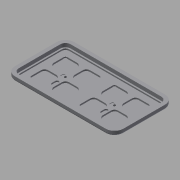
# Autodesk Inventor part: V4 dual
Saved by Autodesk Inventor 2018 (Build 220112000, 112)
## iProperties
Created: 2020-01-08
Part Number: V4 dual
Material: Generic
Document SubType Name: Modeling
Designer: user
Density: 1 g/cm^3
Appearance: Default
Author: user
Autodesk Inventor part; units mm, degrees
ref_plane "YZ Plane" through (0, 0, 0) normal (1, 0, 0) x (0, 1, 0)
ref_plane "XZ Plane" through (0, 0, 0) normal (0, 1, 0) x (-1, 0, 0)
ref_plane "XY Plane" through (0, 0, 0) normal (0, 0, 1) x (1, 0, 0)
sketch "Sketch1" plane through (0, 0, 0) normal (0, 0, 1) x (1, 0, 0)
  line L0 (-62, 40.5) -> (62, 40.5)
  line L1 (74, 28.5) -> (74, -28.5)
  line L2 (62, -40.5) -> (-62, -40.5)
  line L3 (-74, -28.5) -> (-74, 28.5)
  arc A0 (-62, 40.5) -> (-74, 28.5) centre (-62, 28.5) ccw
  arc A1 (74, 28.5) -> (62, 40.5) centre (62, 28.5) ccw
  arc A2 (62, -40.5) -> (74, -28.5) centre (62, -28.5) ccw
  arc A3 (-74, -28.5) -> (-62, -40.5) centre (-62, -28.5) ccw
  line L4 (-62, 28.5) -> (62, -28.5) construction
  point P0 (0, 0)
  point P1 (0, 0)
  dimension "d0" = 12
  dimension "d1" = 81
  dimension "d40" = 148
  constraints: 10 end point, 8 point on circle, 8 tangent, 4 centre point, 3 equal radius, 2 parallel, 1 coincident, 1 horizontal, 1 midpoint, 1 perpendicular
  measures "d0" radius of A0
  measures "d1" distance between parallel lines of L2 L0
  measures "d40" distance between parallel lines of L1 L3
extrude "Extrusion1" add sketch "Sketch1" along normal blind 10.25
sketch "Sketch2" plane through (0, 0, 10.25) normal (0, 0, 1) x (1, 0, 0)
  line L0 (62, 40.5) -> (-62, 40.5) construction
  arc A0 (-62, 40.5) -> (-74, 28.5) centre (-62, 28.5) ccw construction
  line L1 (-74, 28.5) -> (-74, -28.5) construction
  arc A1 (-74, -28.5) -> (-62, -40.5) centre (-62, -28.5) ccw construction
  line L2 (-62, -40.5) -> (62, -40.5) construction
  arc A2 (62, -40.5) -> (74, -28.5) centre (62, -28.5) ccw construction
  line L3 (74, -28.5) -> (74, 28.5) construction
  arc A3 (74, 28.5) -> (62, 40.5) centre (62, 28.5) ccw construction
  line L4 (-62, 35.5) -> (62, 35.5)
  arc A4 (69, 28.5) -> (62, 35.5) centre (62, 28.5) ccw
  line L5 (69, 28.5) -> (69, -28.5)
  arc A5 (62, -35.5) -> (69, -28.5) centre (62, -28.5) ccw
  line L6 (62, -35.5) -> (-62, -35.5)
  arc A6 (-69, -28.5) -> (-62, -35.5) centre (-62, -28.5) ccw
  line L7 (-69, -28.5) -> (-69, 28.5)
  arc A7 (-62, 35.5) -> (-69, 28.5) centre (-62, 28.5) ccw
  point P0 (0, 0)
  dimension "d4" = 5
  constraints: 8 end point, 8 point on circle, 4 centre point, 7 other
  measures "d4" distance between parallel lines of L1 L7
extrude "Extrusion2" cut sketch "Sketch2" against normal blind 5
sketch "Sketch3" plane through (0, 0, 5.25) normal (0, 0, 1) x (1, 0, 0)
  line L0 (-62, 35.5) -> (62, 35.5) construction
  arc A0 (-62, 35.5) -> (-69, 28.5) centre (-62, 28.5) ccw construction
  line L1 (-69, -28.5) -> (-69, 28.5) construction
  arc A1 (-69, -28.5) -> (-62, -35.5) centre (-62, -28.5) ccw construction
  line L2 (62, -35.5) -> (-62, -35.5) construction
  arc A2 (62, -35.5) -> (69, -28.5) centre (62, -28.5) ccw construction
  line L3 (69, 28.5) -> (69, -28.5) construction
  arc A3 (69, 28.5) -> (62, 35.5) centre (62, 28.5) ccw construction
  line L4 (62, 33.5) -> (-62, 33.5)
  arc A4 (-62, 33.5) -> (-67, 28.5) centre (-62, 28.5) ccw
  line L5 (-67, 28.5) -> (-67, -28.5)
  arc A5 (-67, -28.5) -> (-62, -33.5) centre (-62, -28.5) ccw
  line L6 (-62, -33.5) -> (62, -33.5)
  arc A6 (62, -33.5) -> (67, -28.5) centre (62, -28.5) ccw
  line L7 (67, -28.5) -> (67, 28.5)
  arc A7 (67, 28.5) -> (62, 33.5) centre (62, 28.5) ccw
  point P0 (0, 0)
  dimension "d7" = 2
  constraints: 8 end point, 8 point on circle, 4 centre point, 7 other
  measures "d7" distance between parallel lines of L0 L4
extrude "Extrusion3" cut sketch "Sketch3" against normal blind 1.75
chamfer "Chamfer1" distance 9 angle 30 8 edges at (0, 40.5, 0) (70.4853, 36.9853, 0) (74, 0, 0) (70.4853, -36.9853, 0) (0, -40.5, 0) (-70.4853, -36.9853, 0) (-74, 0, 0) (-70.4853, 36.9853, 0) measured on face at (70.1317, 36.6317, 0) measured on face at (0, 40, 0) measured on face at (-70.1317, -36.6317, 0) measured on face at (0, -40, 0) measured on face at (-73.5, 0, 0) measured on face at (70.1317, -36.6317, 0) measured on face at (73.5, 0, 0) measured on face at (-70.1317, 36.6317, 0)
sketch "Sketch5" plane through (0, 0, 0) normal (0, 0, -1) x (-1, 0, 0)
  line L0 (24.75, 3.75) -> (13.75, 3.75)
  line L1 (8.75, 8.75) -> (8.75, 22.0251)
  line L2 (11.4749, 24.75) -> (24.75, 24.75)
  line L3 (29.75, 19.75) -> (29.75, 8.75)
  arc A0 (8.75, 8.75) -> (13.75, 3.75) centre (13.75, 8.75) ccw
  arc A1 (29.75, 19.75) -> (24.75, 24.75) centre (24.75, 19.75) ccw
  arc A2 (24.75, 3.75) -> (29.75, 8.75) centre (24.75, 8.75) ccw
  line L4 (50.752, -17.252) -> (24.75, 8.75) construction
  line L5 (24.75, 24.25) -> (11.4749, 24.25)
  line L6 (9.25, 22.0251) -> (9.25, 8.75)
  arc A3 (9.25, 8.75) -> (13.75, 4.25) centre (13.75, 8.75) ccw
  line L7 (13.75, 4.25) -> (24.75, 4.25)
  arc A4 (24.75, 4.25) -> (29.25, 8.75) centre (24.75, 8.75) ccw
  line L8 (29.25, 8.75) -> (29.25, 19.75)
  arc A5 (29.25, 19.75) -> (24.75, 24.25) centre (24.75, 19.75) ccw
  line L9 (-12.252, 45.752) -> (13.75, 19.75) construction
  line L10 (24.75, 24.25) -> (24.75, 4.25) construction
  line L11 (9.25, 8.75) -> (29.25, 8.75) construction
  line L12 (24.75, 24.25) -> (24.75, 24.75) construction
  line L13 (9.25, 8.75) -> (8.75, 8.75) construction
  line L14 (24.75, 19.75) -> (13.75, 19.75) construction
  line L15 (13.75, 8.75) -> (13.75, 19.75) construction
  arc A6 (11.2249, 24.5) -> (11.4749, 24.25) centre (11.4749, 24.5) ccw
  arc A7 (11.4749, 24.75) -> (11.2249, 24.5) centre (11.4749, 24.5) ccw
  arc A8 (9.25, 22.0251) -> (9, 21.7751) centre (9, 22.0251) ccw construction
  arc A9 (9, 21.7751) -> (8.75, 22.0251) centre (9, 22.0251) ccw construction
  line L16 (10.2374, 23.2626) -> (11.2981, 24.3232) construction
  line L17 (10.2374, 23.2626) -> (9.1768, 22.2019) construction
  arc A10 (-62, 31.5) -> (-65, 28.5) centre (-62, 28.5) ccw construction
  arc A11 (9.25, 22.0251) -> (8.75, 22.0251) centre (9, 22.0251) ccw
  line L18 (29.75, -8.75) -> (29.75, -19.75)
  line L19 (24.75, -4.25) -> (13.75, -4.25)
  line L20 (29.25, -19.75) -> (29.25, -8.75)
  line L21 (9.25, -8.75) -> (29.25, -8.75) construction
  line L22 (24.75, -24.25) -> (24.75, -4.25) construction
  arc A12 (13.75, -4.25) -> (9.25, -8.75) centre (13.75, -8.75) ccw
  line L23 (24.75, -19.75) -> (13.75, -19.75) construction
  line L24 (13.75, -8.75) -> (13.75, -19.75) construction
  line L25 (10.2374, -23.2626) -> (11.2981, -24.3232) construction
  line L26 (9.25, -8.75) -> (9.25, -22.0251)
  line L27 (8.75, -22.0251) -> (8.75, -8.75)
  line L28 (9.25, -8.75) -> (8.75, -8.75) construction
  arc A13 (13.75, -3.75) -> (8.75, -8.75) centre (13.75, -8.75) ccw
  line L29 (13.75, -3.75) -> (24.75, -3.75)
  arc A14 (29.75, -8.75) -> (24.75, -3.75) centre (24.75, -8.75) ccw
  arc A15 (29.25, -8.75) -> (24.75, -4.25) centre (24.75, -8.75) ccw
  line L30 (24.75, -24.75) -> (11.4749, -24.75)
  line L31 (11.4749, -24.25) -> (24.75, -24.25)
  line L32 (24.75, -24.25) -> (24.75, -24.75) construction
  arc A16 (24.75, -24.25) -> (29.25, -19.75) centre (24.75, -19.75) ccw
  arc A17 (24.75, -24.75) -> (29.75, -19.75) centre (24.75, -19.75) ccw
  arc A18 (8.75, -22.0251) -> (9, -22.2751) centre (9, -22.0251) ccw
  arc A19 (9, -22.2751) -> (9.25, -22.0251) centre (9, -22.0251) ccw
  line L33 (10.2374, -23.2626) -> (9.1768, -22.2019) construction
  arc A20 (11.7249, -24.5) -> (11.4749, -24.75) centre (11.4749, -24.5) ccw construction
  arc A21 (11.4749, -24.25) -> (11.7249, -24.5) centre (11.4749, -24.5) ccw construction
  arc A22 (11.4749, -24.25) -> (11.4749, -24.75) centre (11.4749, -24.5) ccw
  line L34 (42.25, -3.75) -> (53.25, -3.75)
  line L35 (37.75, -8.75) -> (37.75, -19.75)
  line L36 (53.25, -4.25) -> (42.25, -4.25)
  line L37 (42.25, -24.25) -> (42.25, -4.25) construction
  line L38 (57.75, -8.75) -> (37.75, -8.75) construction
  arc A23 (37.75, -19.75) -> (42.25, -24.25) centre (42.25, -19.75) ccw
  line L39 (53.25, -8.75) -> (53.25, -19.75) construction
  line L40 (42.25, -19.75) -> (53.25, -19.75) construction
  line L41 (56.7626, -23.2626) -> (57.8232, -22.2019) construction
  line L42 (42.25, -24.25) -> (55.5251, -24.25)
  line L43 (55.5251, -24.75) -> (42.25, -24.75)
  line L44 (42.25, -24.25) -> (42.25, -24.75) construction
  arc A24 (37.25, -19.75) -> (42.25, -24.75) centre (42.25, -19.75) ccw
  line L45 (37.25, -19.75) -> (37.25, -8.75)
  arc A25 (42.25, -3.75) -> (37.25, -8.75) centre (42.25, -8.75) ccw
  arc A26 (42.25, -4.25) -> (37.75, -8.75) centre (42.25, -8.75) ccw
  line L46 (58.25, -8.75) -> (58.25, -22.0251)
  line L47 (57.75, -22.0251) -> (57.75, -8.75)
  line L48 (57.75, -8.75) -> (58.25, -8.75) construction
  arc A27 (57.75, -8.75) -> (53.25, -4.25) centre (53.25, -8.75) ccw
  arc A28 (58.25, -8.75) -> (53.25, -3.75) centre (53.25, -8.75) ccw
  arc A29 (55.5251, -24.75) -> (55.7751, -24.5) centre (55.5251, -24.5) ccw
  arc A30 (55.7751, -24.5) -> (55.5251, -24.25) centre (55.5251, -24.5) ccw
  line L49 (56.7626, -23.2626) -> (55.7019, -24.3232) construction
  arc A31 (58, -21.7751) -> (58.25, -22.0251) centre (58, -22.0251) ccw construction
  arc A32 (57.75, -22.0251) -> (58, -21.7751) centre (58, -22.0251) ccw construction
  arc A33 (57.75, -22.0251) -> (58.25, -22.0251) centre (58, -22.0251) ccw
  line L50 (37.25, 8.75) -> (37.25, 19.75)
  line L51 (42.25, 4.25) -> (53.25, 4.25)
  line L52 (37.75, 19.75) -> (37.75, 8.75)
  line L53 (57.75, 8.75) -> (37.75, 8.75) construction
  line L54 (42.25, 24.25) -> (42.25, 4.25) construction
  arc A34 (53.25, 4.25) -> (57.75, 8.75) centre (53.25, 8.75) ccw
  line L55 (42.25, 19.75) -> (53.25, 19.75) construction
  line L56 (53.25, 8.75) -> (53.25, 19.75) construction
  line L57 (56.7626, 23.2626) -> (55.7019, 24.3232) construction
  line L58 (57.75, 8.75) -> (57.75, 22.0251)
  line L59 (58.25, 22.0251) -> (58.25, 8.75)
  line L60 (57.75, 8.75) -> (58.25, 8.75) construction
  arc A35 (53.25, 3.75) -> (58.25, 8.75) centre (53.25, 8.75) ccw
  line L61 (53.25, 3.75) -> (42.25, 3.75)
  arc A36 (37.25, 8.75) -> (42.25, 3.75) centre (42.25, 8.75) ccw
  arc A37 (37.75, 8.75) -> (42.25, 4.25) centre (42.25, 8.75) ccw
  line L62 (42.25, 24.75) -> (55.5251, 24.75)
  line L63 (55.5251, 24.25) -> (42.25, 24.25)
  line L64 (42.25, 24.25) -> (42.25, 24.75) construction
  arc A38 (42.25, 24.25) -> (37.75, 19.75) centre (42.25, 19.75) ccw
  arc A39 (42.25, 24.75) -> (37.25, 19.75) centre (42.25, 19.75) ccw
  arc A40 (58.25, 22.0251) -> (58, 22.2751) centre (58, 22.0251) ccw
  arc A41 (58, 22.2751) -> (57.75, 22.0251) centre (58, 22.0251) ccw
  line L65 (56.7626, 23.2626) -> (57.8232, 22.2019) construction
  arc A42 (55.2751, 24.5) -> (55.5251, 24.75) centre (55.5251, 24.5) ccw construction
  arc A43 (55.5251, 24.25) -> (55.2751, 24.5) centre (55.5251, 24.5) ccw construction
  arc A44 (55.5251, 24.25) -> (55.5251, 24.75) centre (55.5251, 24.5) ccw
  line L66 (33.5, 0) -> (0, 0)
  line L67 (58.25, -15.3876) -> (65, -15.3876) construction
  line L68 (65, 28.5) -> (65, -28.5) construction
  line L69 (48.8876, -24.75) -> (48.8876, -31.5) construction
  line L70 (62, -31.5) -> (-62, -31.5) construction
  point P0 (11.2249, 24.75)
  point P1 (8.75, 21.7751)
  point P2 (9.25, 21.7751)
  point P3 (11.2249, 24.25)
  point P4 (9.25, -22.2751)
  point P5 (8.75, -22.2751)
  point P6 (11.7249, -24.75)
  point P7 (11.7249, -24.25)
  point P8 (55.7751, -24.25)
  point P9 (55.7751, -24.75)
  point P10 (58.25, -21.7751)
  point P11 (57.75, -21.7751)
  point P12 (57.75, 22.2751)
  point P13 (58.25, 22.2751)
  point P14 (55.2751, 24.75)
  point P15 (55.2751, 24.25)
  dimension "d23" = 0.5
  dimension "d24" = 5
  dimension "d25" = 20
  dimension "d26" = 0.25
  dimension "d27" = 3
  dimension "d32" = 360
  dimension "d41" = 7.5
  constraints: 138 end point, 96 point on circle, 44 centre point, 27 point on line, 11 tangent, 7 perpendicular, 6 equal length, 4 horizontal, 4 parallel, 3 collinear, 3 equal radius, 2 midpoint, 2 vertical, 1 coincident, 315 other
  measures "d23" distance between parallel lines of L0 L7
  measures "d24" radius of A0
  measures "d25" distance between parallel lines of L8 L6
  measures "d26" radius of A6
  measures "d27" distance of L17.end L16.end
  measures "d41" distance between parallel lines of L50 L3
extrude "Extrusion4" cut sketch "Sketch5" against normal through all
fillet "Fillet2" radius 2 16 edges at (70.4853, 36.9853, 5.1962) (74, 0, 5.1962) (70.4853, -36.9853, 5.1962) (0, -40.5, 5.1962) (-70.4853, -36.9853, 5.1962) (-74, 0, 5.1962) (-70.4853, 36.9853, 5.1962) (0, 40.5, 5.1962) (-64.1213, 30.6213, 0) (-65, 0, 0) (-64.1213, -30.6213, 0) (0, -31.5, 0) (64.1213, -30.6213, 0) (65, 0, 0) (64.1213, 30.6213, 0) (0, 31.5, 0)
sketch "Sketch7" plane through (0, 0, 3.5) normal (0, 0, 1) x (1, 0, 0)
  line L0 (-37.25, -8.75) -> (-37.25, -19.75) projected
  arc A0 (-42.25, -24.75) -> (-37.25, -19.75) centre (-42.25, -19.75) ccw projected
  line L1 (-42.25, -24.75) -> (-55.5251, -24.75) projected
  arc A1 (-55.5251, -24.25) -> (-55.5251, -24.75) centre (-55.5251, -24.5) ccw projected
  line L2 (-55.5251, -24.25) -> (-42.25, -24.25) projected
  arc A2 (-42.25, -24.25) -> (-37.75, -19.75) centre (-42.25, -19.75) ccw projected
  line L3 (-37.75, -19.75) -> (-37.75, -8.75) projected
  arc A3 (-37.75, -8.75) -> (-42.25, -4.25) centre (-42.25, -8.75) ccw projected
  line L4 (-42.25, -4.25) -> (-53.25, -4.25) projected
  arc A4 (-53.25, -4.25) -> (-57.75, -8.75) centre (-53.25, -8.75) ccw projected
  line L5 (-57.75, -8.75) -> (-57.75, -22.0251) projected
  arc A5 (-58.25, -22.0251) -> (-57.75, -22.0251) centre (-58, -22.0251) ccw projected
  line L6 (-58.25, -22.0251) -> (-58.25, -8.75) projected
  arc A6 (-53.25, -3.75) -> (-58.25, -8.75) centre (-53.25, -8.75) ccw projected
  line L7 (-53.25, -3.75) -> (-42.25, -3.75) projected
  arc A7 (-37.25, -8.75) -> (-42.25, -3.75) centre (-42.25, -8.75) ccw projected
  line L8 (-11.4749, 24.25) -> (-24.75, 24.25) projected
  arc A8 (-24.75, 24.25) -> (-29.25, 19.75) centre (-24.75, 19.75) ccw projected
  line L9 (-29.25, 19.75) -> (-29.25, 8.75) projected
  arc A9 (-29.25, 8.75) -> (-24.75, 4.25) centre (-24.75, 8.75) ccw projected
  line L10 (-24.75, 4.25) -> (-13.75, 4.25) projected
  arc A10 (-13.75, 4.25) -> (-9.25, 8.75) centre (-13.75, 8.75) ccw projected
  line L11 (-9.25, 8.75) -> (-9.25, 22.0251) projected
  arc A11 (-8.75, 22.0251) -> (-9.25, 22.0251) centre (-9, 22.0251) ccw projected
  line L12 (-8.75, 22.0251) -> (-8.75, 8.75) projected
  arc A12 (-13.75, 3.75) -> (-8.75, 8.75) centre (-13.75, 8.75) ccw projected
  line L13 (-13.75, 3.75) -> (-24.75, 3.75) projected
  arc A13 (-29.75, 8.75) -> (-24.75, 3.75) centre (-24.75, 8.75) ccw projected
  line L14 (-29.75, 8.75) -> (-29.75, 19.75) projected
  arc A14 (-24.75, 24.75) -> (-29.75, 19.75) centre (-24.75, 19.75) ccw projected
  line L15 (-24.75, 24.75) -> (-11.4749, 24.75) projected
  arc A15 (-11.4749, 24.25) -> (-11.4749, 24.75) centre (-11.4749, 24.5) ccw projected
  line L16 (-24.75, -3.75) -> (-13.75, -3.75) projected
  arc A16 (-8.75, -8.75) -> (-13.75, -3.75) centre (-13.75, -8.75) ccw projected
  line L17 (-8.75, -8.75) -> (-8.75, -22.0251) projected
  arc A17 (-9.25, -22.0251) -> (-8.75, -22.0251) centre (-9, -22.0251) ccw projected
  line L18 (-9.25, -22.0251) -> (-9.25, -8.75) projected
  arc A18 (-9.25, -8.75) -> (-13.75, -4.25) centre (-13.75, -8.75) ccw projected
  line L19 (-13.75, -4.25) -> (-24.75, -4.25) projected
  arc A19 (-24.75, -4.25) -> (-29.25, -8.75) centre (-24.75, -8.75) ccw projected
  line L20 (-29.25, -8.75) -> (-29.25, -19.75) projected
  arc A20 (-29.25, -19.75) -> (-24.75, -24.25) centre (-24.75, -19.75) ccw projected
  line L21 (-24.75, -24.25) -> (-11.4749, -24.25) projected
  arc A21 (-11.4749, -24.75) -> (-11.4749, -24.25) centre (-11.4749, -24.5) ccw projected
  line L22 (-11.4749, -24.75) -> (-24.75, -24.75) projected
  arc A22 (-29.75, -19.75) -> (-24.75, -24.75) centre (-24.75, -19.75) ccw projected
  line L23 (-29.75, -19.75) -> (-29.75, -8.75) projected
  arc A23 (-24.75, -3.75) -> (-29.75, -8.75) centre (-24.75, -8.75) ccw projected
  line L24 (-42.25, 3.75) -> (-53.25, 3.75) projected
  arc A24 (-58.25, 8.75) -> (-53.25, 3.75) centre (-53.25, 8.75) ccw projected
  line L25 (-58.25, 8.75) -> (-58.25, 22.0251) projected
  arc A25 (-57.75, 22.0251) -> (-58.25, 22.0251) centre (-58, 22.0251) ccw projected
  line L26 (-57.75, 22.0251) -> (-57.75, 8.75) projected
  arc A26 (-57.75, 8.75) -> (-53.25, 4.25) centre (-53.25, 8.75) ccw projected
  line L27 (-53.25, 4.25) -> (-42.25, 4.25) projected
  arc A27 (-42.25, 4.25) -> (-37.75, 8.75) centre (-42.25, 8.75) ccw projected
  line L28 (-37.75, 8.75) -> (-37.75, 19.75) projected
  arc A28 (-37.75, 19.75) -> (-42.25, 24.25) centre (-42.25, 19.75) ccw projected
  line L29 (-42.25, 24.25) -> (-55.5251, 24.25) projected
  arc A29 (-55.5251, 24.75) -> (-55.5251, 24.25) centre (-55.5251, 24.5) ccw projected
  line L30 (-55.5251, 24.75) -> (-42.25, 24.75) projected
  arc A30 (-37.25, 19.75) -> (-42.25, 24.75) centre (-42.25, 19.75) ccw projected
  line L31 (-37.25, 19.75) -> (-37.25, 8.75) projected
  arc A31 (-42.25, 3.75) -> (-37.25, 8.75) centre (-42.25, 8.75) ccw projected
  line L32 (-62, 33.5) -> (62, 33.5) projected
  arc A32 (-62, 33.5) -> (-67, 28.5) centre (-62, 28.5) ccw projected
  line L33 (-67, -28.5) -> (-67, 28.5) projected
  arc A33 (-67, -28.5) -> (-62, -33.5) centre (-62, -28.5) ccw projected
  line L34 (62, -33.5) -> (-62, -33.5) projected
  arc A34 (62, -33.5) -> (67, -28.5) centre (62, -28.5) ccw projected
  line L35 (67, 28.5) -> (67, -28.5) projected
  arc A35 (67, 28.5) -> (62, 33.5) centre (62, 28.5) ccw projected
  arc A36 (-58.25, -22.0251) -> (-55.5251, -24.75) centre (-55.5251, -22.0251) ccw
  arc A37 (-55.5251, 24.75) -> (-58.25, 22.0251) centre (-55.5251, 22.0251) ccw
  arc A38 (-11.4749, 24.25) -> (-11.4749, 24.75) centre (-11.4749, 24.5) ccw projected
  arc A39 (-8.75, 22.0251) -> (-11.4749, 24.75) centre (-11.4749, 22.0251) ccw
  line L36 (-11.4749, -24.75) -> (-24.75, -24.75) projected
  arc A40 (-11.4749, -24.75) -> (-8.75, -22.0251) centre (-11.4749, -22.0251) ccw
  point P0 (0, 0)
  constraints: 8 point on circle, 4 centre point, 4 tangent
extrude "Extrusion6" cut sketch "Sketch7" against normal blind 1.5 contours L0 A0 L1 A1 L2 A2 L3 A3 L4 A4 L5 A5 L6 A6 L7 A7 | A36 A5 L5 A4 L4 A3 L3 A2 L2 A1 | A15 A39 A11 L11 A10 L10 A9 L9 A8 L8 | L8 A8 L9 A9 L10 A10 L11 A11 L12 A12 L13 A13 L14 A14 L15 A15 | L16 A16 L17 A17 L18 A18 L19 A19 L20 A20 L21 A21 L22 A22 L23 A23 | A40 A21 L21 A20 L20 A19 L19 A18 L18 A17 | L24 A24 L25 A25 L26 A26 L27 A27 L28 A28 L29 A29 L30 A30 L31 A31 | A37 A29 L29 A28 L28 A27 L27 A26 L26 A25
sketch "Sketch8" plane through (0, 0, 0) normal (0, 0, -1) x (-1, 0, 0)
  arc A0 (42.25, -4.25) -> (37.75, -8.75) centre (42.25, -8.75) ccw construction
  arc A1 (24.75, 4.25) -> (29.25, 8.75) centre (24.75, 8.75) ccw construction
  line L0 (42.25, -8.75) -> (24.75, 8.75) construction
  point P0 (0, 0)
  point P1 (33.5, 0)
  constraints: 2 end point, 1 midpoint
hole "Hole1" at (-33.5, 0, 0) direction (0, 0, 1) diameter 3.2 end through all counterbore diameter 5.7 counterbore depth 2.7
sketch "Sketch10" plane through (0, 0, 3.5) normal (0, 0, 1) x (1, 0, 0)
  line L0 (-37.961, -2.5) -> (-36.461, -2.5)
  line L1 (-35.711, -1.75) -> (-35.711, 1.75)
  line L2 (-36.461, 2.5) -> (-37.961, 2.5)
  line L3 (-38.711, 1.75) -> (-38.711, -1.75)
  line L4 (-33.5, -16.4884) -> (-33.5, -11.4084) construction
  line L5 (-31.25, -16.4884) -> (-31.25, -11.4084)
  line L6 (-35.75, -11.4084) -> (-35.75, -16.4884)
  arc A0 (-35.75, -16.4884) -> (-31.25, -16.4884) centre (-33.5, -16.4884) ccw
  arc A1 (-31.25, -11.4084) -> (-35.75, -11.4084) centre (-33.5, -11.4084) ccw
  circle A2 centre (-33.5, 0) radius 1.6 construction
  line L7 (-35.75, -13.9484) -> (-35.75, -12.4484) construction
  line L8 (-31.25, -13.9484) -> (-31.25, -15.4484) construction
  arc A3 (-37.961, 2.5) -> (-38.711, 1.75) centre (-37.961, 1.75) ccw
  arc A4 (-38.711, -1.75) -> (-37.961, -2.5) centre (-37.961, -1.75) ccw
  arc A5 (-36.461, -2.5) -> (-35.711, -1.75) centre (-36.461, -1.75) ccw
  arc A6 (-35.711, 1.75) -> (-36.461, 2.5) centre (-36.461, 1.75) ccw
  line L9 (-37.961, -1.75) -> (-33.5, 0) construction
  line L10 (-33.5, 0) -> (-37.961, 1.75) construction
  line L11 (-37.25, -8.75) -> (-37.25, -19.75) construction
  point P0 (-38.711, -2.5)
  point P1 (-35.711, 2.5)
  point P2 (-38.711, 2.5)
  point P3 (-33.5, -13.9484)
  dimension "d70" = 5
  dimension "d71" = 3
  dimension "d73" = 5.08
  dimension "d76" = 0.75
  dimension "d84" = 13.9484
  dimension "d85" = 2.211
  dimension "d86" = 4.5
  constraints: 24 end point, 12 point on circle, 12 tangent, 7 point on line, 6 centre point, 5 parallel, 3 equal radius, 3 midpoint, 2 coincident, 2 equal length, 1 perpendicular
  measures "d70" distance of point (-38.711, 2.5) point (-38.711, -2.5)
  measures "d71" distance of point (-35.711, 2.5) point (-38.711, 2.5)
  measures "d73" distance of L5.start L5.end
  measures "d76" radius of A3
  measures "d84" distance of L9.end point (-33.5, -13.948)
  measures "d85" distance from line of L9.end L1
  measures "d86" distance between parallel lines of L5 L6
extrude "Extrusion7" cut sketch "Sketch10" against normal blind 0.64 contours A4 L3 A3 L2 A6 L1 A5 L0
extrude "Extrusion8" cut sketch "Sketch10" against normal blind 1.75 contours A0 L6 A1 L5
sketch "Sketch9" plane through (0, 0, 0) normal (0, 0, -1) x (-1, 0, 0)
  arc A0 (29.25, 19.75) -> (24.75, 24.25) centre (24.75, 19.75) ccw construction
  circle A1 centre (33.5, 0) radius 1.6 construction
  arc A2 (9.25, 8.75) -> (13.75, 4.25) centre (13.75, 8.75) ccw construction
  line L0 (24.75, 19.75) -> (13.75, 8.75) construction
  circle A3 centre (19.25, 14.25) radius 2
  circle A4 centre (16.4216, 11.4216) radius 2
  circle A5 centre (17.25, 10.7859) radius 2
  circle A6 centre (18.2147, 10.3863) radius 2
  circle A7 centre (19.25, 10.25) radius 2
  circle A8 centre (20.2853, 10.3863) radius 2
  circle A9 centre (21.25, 10.7859) radius 2
  circle A10 centre (22.0784, 11.4216) radius 2
  circle A11 centre (22.7141, 12.25) radius 2
  circle A12 centre (23.1137, 13.2147) radius 2
  circle A13 centre (23.25, 14.25) radius 2
  circle A14 centre (23.1137, 15.2853) radius 2
  circle A15 centre (22.7141, 16.25) radius 2
  circle A16 centre (22.0784, 17.0784) radius 2
  circle A17 centre (21.25, 17.7141) radius 2
  circle A18 centre (20.2853, 18.1137) radius 2
  circle A19 centre (19.25, 18.25) radius 2
  circle A20 centre (18.2147, 18.1137) radius 2
  circle A21 centre (17.25, 17.7141) radius 2
  circle A22 centre (16.4216, 17.0784) radius 2
  circle A23 centre (15.7859, 16.25) radius 2
  circle A24 centre (15.3863, 15.2853) radius 2
  circle A25 centre (15.25, 14.25) radius 2
  circle A26 centre (15.3863, 13.2147) radius 2
  circle A27 centre (15.7859, 12.25) radius 2
  circle A28 centre (22.7141, -12.25) radius 2
  circle A29 centre (23.1137, -13.2147) radius 2
  circle A30 centre (23.1137, -15.2853) radius 2
  circle A31 centre (22.7141, -16.25) radius 2
  circle A32 centre (23.25, -14.25) radius 2
  circle A33 centre (15.3863, -13.2147) radius 2
  circle A34 centre (15.25, -14.25) radius 2
  circle A35 centre (15.3863, -15.2853) radius 2
  circle A36 centre (19.25, -18.25) radius 2
  circle A37 centre (18.2147, -18.1137) radius 2
  circle A38 centre (15.7859, -16.25) radius 2
  circle A39 centre (16.4216, -17.0784) radius 2
  circle A40 centre (17.25, -17.7141) radius 2
  circle A41 centre (22.0784, -11.4216) radius 2
  circle A42 centre (21.25, -10.7859) radius 2
  line L1 (13.75, -8.75) -> (24.75, -19.75) construction
  circle A43 centre (19.25, -14.25) radius 2
  circle A44 centre (19.25, -10.25) radius 2
  circle A45 centre (15.7859, -12.25) radius 2
  circle A46 centre (18.2147, -10.3863) radius 2
  circle A47 centre (16.4216, -11.4216) radius 2
  circle A48 centre (17.25, -10.7859) radius 2
  circle A49 centre (20.2853, -10.3863) radius 2
  circle A50 centre (22.0784, -17.0784) radius 2
  circle A51 centre (20.2853, -18.1137) radius 2
  circle A52 centre (21.25, -17.7141) radius 2
  circle A53 centre (45.75, -10.7859) radius 2
  circle A54 centre (46.7147, -10.3863) radius 2
  circle A55 centre (48.7853, -10.3863) radius 2
  circle A56 centre (49.75, -10.7859) radius 2
  circle A57 centre (47.75, -10.25) radius 2
  circle A58 centre (46.7147, -18.1137) radius 2
  circle A59 centre (47.75, -18.25) radius 2
  circle A60 centre (48.7853, -18.1137) radius 2
  circle A61 centre (51.75, -14.25) radius 2
  circle A62 centre (51.6137, -15.2853) radius 2
  circle A63 centre (49.75, -17.7141) radius 2
  circle A64 centre (50.5784, -17.0784) radius 2
  circle A65 centre (51.2141, -16.25) radius 2
  circle A66 centre (44.9216, -11.4216) radius 2
  circle A67 centre (44.2859, -12.25) radius 2
  line L2 (42.25, -19.75) -> (53.25, -8.75) construction
  circle A68 centre (47.75, -14.25) radius 2
  circle A69 centre (43.75, -14.25) radius 2
  circle A70 centre (45.75, -17.7141) radius 2
  circle A71 centre (43.8863, -15.2853) radius 2
  circle A72 centre (44.9216, -17.0784) radius 2
  circle A73 centre (44.2859, -16.25) radius 2
  circle A74 centre (43.8863, -13.2147) radius 2
  circle A75 centre (50.5784, -11.4216) radius 2
  circle A76 centre (51.6137, -13.2147) radius 2
  circle A77 centre (51.2141, -12.25) radius 2
  circle A78 centre (44.2859, 12.25) radius 2
  circle A79 centre (43.8863, 13.2147) radius 2
  circle A80 centre (43.8863, 15.2853) radius 2
  circle A81 centre (44.2859, 16.25) radius 2
  circle A82 centre (43.75, 14.25) radius 2
  circle A83 centre (51.6137, 13.2147) radius 2
  circle A84 centre (51.75, 14.25) radius 2
  circle A85 centre (51.6137, 15.2853) radius 2
  circle A86 centre (47.75, 18.25) radius 2
  circle A87 centre (48.7853, 18.1137) radius 2
  circle A88 centre (51.2141, 16.25) radius 2
  circle A89 centre (50.5784, 17.0784) radius 2
  circle A90 centre (49.75, 17.7141) radius 2
  circle A91 centre (44.9216, 11.4216) radius 2
  circle A92 centre (45.75, 10.7859) radius 2
  line L3 (53.25, 8.75) -> (42.25, 19.75) construction
  circle A93 centre (47.75, 14.25) radius 2
  circle A94 centre (47.75, 10.25) radius 2
  circle A95 centre (51.2141, 12.25) radius 2
  circle A96 centre (48.7853, 10.3863) radius 2
  circle A97 centre (50.5784, 11.4216) radius 2
  circle A98 centre (49.75, 10.7859) radius 2
  circle A99 centre (46.7147, 10.3863) radius 2
  circle A100 centre (44.9216, 17.0784) radius 2
  circle A101 centre (46.7147, 18.1137) radius 2
  circle A102 centre (45.75, 17.7141) radius 2
  point P0 (0, 0)
  dimension "d58" = 4
  dimension "d61" = 360
  dimension "d65" = 360
  constraints: 101 centre point, 8 end point, 4 point on line, 2 equal radius, 2 point on circle, 1 midpoint, 262 other
  measures "d58" diameter of A3
emboss "Emboss1" sketch "Sketch9" operation add depth 0.5 direction (0, 0, 1) contours A16 A17 A15 | A15 A17 A14 A16 | A14 A17 A13 A16 | A10 A11 A9 | A10 A12 A9 A11 | A10 A13 A9 A12 | A13 A16 | A10 A13 | A16 A18 A15 A17 | A15 A18 A14 A17 | A14 A17 | A9 A11 A8 A10 | A9 A12 A8 A11 | A9 A12 | A17 A14 A16 A13 | A13 A10 A12 A9 | A16 A19 A15 A18 | A15 A18 | A18 A15 A17 A14 | A8 A11 A7 A10 | A8 A11 | A12 A9 A11 A8 | A17 A15 A16 A14 | A12 A10 A11 A9 | A16 A19 | A19 A16 A18 A15 | A7 A10 | A11 A8 A10 A7 | A18 A16 A17 A15 | A11 A9 A10 A8 | A17 A16 A15 | A11 A10 A9 | A22 A23 A21 | A21 A23 A20 A22 | A20 A23 A19 A22 | A19 A22 | A4 A5 A27 | A4 A6 A27 A5 | A4 A7 A27 A6 | A4 A7 | A22 A24 A21 A23 | A21 A24 A20 A23 | A20 A23 | A23 A20 A22 A19 | A27 A5 A26 A4 | A27 A6 A26 A5 | A27 A6 | A7 A4 A6 A27 | A22 A25 A21 A24 | A21 A24 | A24 A21 A23 A20 | A23 A21 A22 A20 | A26 A5 A25 A4 | A26 A5 | A6 A27 A5 A26 | A6 A4 A5 A27 | A22 A25 | A25 A22 A24 A21 | A24 A22 A23 A21 | A23 A22 A21 | A25 A4 | A5 A26 A4 A25 | A5 A27 A4 A26 | A5 A4 A27 | A44 A41 | A41 A46 A42 A44 | A42 A46 A49 A44 | A49 A46 A44 | A44 A42 A46 A41 | A46 A42 | A42 A48 A49 A46 | A46 A49 A48 A44 | A44 A49 A46 A42 | A46 A49 A48 A42 | A48 A49 | A48 A49 A47 A44 | A44 A46 A49 | A46 A44 A48 A49 | A48 A44 A47 A49 | A47 A44 | A36 A50 | A36 A52 A37 A50 | A51 A37 A52 A36 | A36 A37 A51 | A36 A51 A37 | A36 A52 A37 A51 | A36 A50 A37 A52 | A37 A52 | A36 A40 A51 A37 | A51 A40 A52 A37 | A37 A51 A40 A36 | A37 A52 A40 A51 | A36 A39 A51 A40 | A51 A40 | A40 A51 A39 A36 | A36 A39 | A68 | A78 A99 | A78 A99 A91 A94 | A99 A79 A92 A78 | A78 A92 A91 A99 | A94 A91 A99 A78 | A94 A91 | A99 A92 A94 A91 | A91 A92 A99 | A99 A78 A92 A79 | A79 A92 | A99 A91 A92 A78 | A94 A92 A96 A91 | A94 A92 A99 A91 | A91 A96 A92 A94 | A99 A92 A91 | A96 A92 | A102 A80 | A102 A80 A101 A81 | A81 A101 A100 A102 | A102 A100 A101 | A102 A81 A101 A80 | A102 A100 A101 A81 | A102 A101 A100 | A101 A81 | A81 A86 A100 A101 | A101 A100 A86 A102 | A84 A85 A83 | A83 A85 A95 A84 | A95 A85 A97 A84 | A97 A84 | A101 A100 A86 A81 | A101 A102 A86 A100 | A97 A85 A95 A84 | A84 A95 A85 A83 | A83 A85 A84 | A86 A100 A87 A102 | A86 A100 | A85 A84 A88 A83 | A83 A88 A95 A85 | A95 A85 | A86 A102 A87 A100 | A85 A95 A88 A83 | A83 A88 A84 A85 | A87 A102 | A88 A84 A89 A83 | A83 A88 | A83 A89 A84 A88 | A89 A84
pattern_linear "Rectangular Pattern1" count 2 spacing 67 along (1, 0, 0) of "Extrusion4", "Extrusion6", "Extrusion7", "Extrusion8", "Emboss1", "Hole1"
pattern_linear "Rectangular Pattern2" count 2 spacing 67 along (1, 0, 0) of "Emboss1"
equation "\"d26\" = 0.5 * d23"
body "Solid1"
